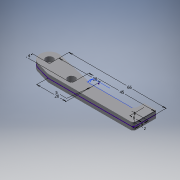
# Autodesk Inventor part: tappy
Saved by Autodesk Inventor 2018 (Build 220112000, 112)
## iProperties
Created: 2018-12-03
Part Number: tappy
Material: Generic
Document SubType Name: Modeling
Designer: Jerry
Density: 1 g/cm^3
Appearance: Default
Author: Jerry
Autodesk Inventor part; units mm, degrees
ref_plane "YZ Plane" through (0, 0, 0) normal (1, 0, 0) x (0, 1, 0)
ref_plane "XZ Plane" through (0, 0, 0) normal (0, 1, 0) x (-1, 0, 0)
ref_plane "XY Plane" through (0, 0, 0) normal (0, 0, 1) x (1, 0, 0)
sketch "Sketch1" plane through (0, 0, 0) normal (0, 0, 1) x (1, 0, 0)
  line L0 (1.4872, 6.2793) -> (27.4317, 0.1346)
  line L1 (28.584, 0) -> (56, 0)
  line L2 (58, 2) -> (58, 6.4531)
  line L3 (58, 6.4531) -> (66, 6.4531)
  line L4 (66, 6.4531) -> (66, -7)
  line L5 (64, -9) -> (8.701, -9)
  line L6 (7.326, -8.8072) -> (-1.7746, -6.2043)
  arc A0 (1.4872, 6.2793) -> (-1.7746, -6.2043) centre (0, 0) ccw
  arc A1 (27.4317, 0.1346) -> (28.584, 0) centre (28.584, 5) ccw
  arc A2 (7.326, -8.8072) -> (8.701, -9) centre (8.701, -4) ccw
  arc A3 (56, 0) -> (58, 2) centre (56, 2) ccw
  arc A4 (64, -9) -> (66, -7) centre (64, -7) ccw
  point P0 (28, 0)
  point P1 (66, -9)
  point P2 (8, -9)
  point P3 (19, -4)
  dimension "d0" = 66
  dimension "d1" = 8
  dimension "d2" = 9
  dimension "d3" = 20
  dimension "d4" = 28
  dimension "d5" = 5
  dimension "d6" = 2
  dimension "d17" = 45
  dimension "d18" = 4
  constraints: 14 end point, 11 tangent, 10 point on circle, 7 point on line, 5 centre point, 4 perpendicular, 2 equal radius, 1 coincident, 1 horizontal, 1 horizontal alignment
  measures "d0" distance from line of L4 A0.centre
  measures "d1" distance of L2.end L3.end
  measures "d2" distance between parallel lines of L1 L5
  measures "d3" horizontal distance of point (28, 0) point (8, -9)
  measures "d4" distance of point (28, 0) point (0, 0)
  measures "d5" radius of A1
  measures "d6" radius of A3
  measures "d17" horizontal distance of A4.centre point (19, -4)
  measures "d18" vertical distance of point (0, 0) point (19, -4)
extrude "Extrusion1" add sketch "Sketch1" along normal mid plane 5
hole "Hole2" at (19, -4, 0) at (0, 0, 0) direction (0, 0, -1) diameter 5.159 end through all both
body "Solid1"
